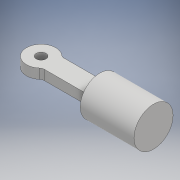
# Autodesk Inventor part: поршень
Saved by Autodesk Inventor 2017.3 (Build 213256000, 256)
## iProperties
Part Number: поршень
Material: Типовые
Document SubType Name: Modeling
Designer: Alexnav
Density: 1 g/cm^3
Appearance: По умолчанию
Mass: 116.064 g
Surface Area: 174.829 cm^2
Volume: 116.064 cm^3
Author: Alexnav
Autodesk Inventor part; units mm, degrees
ref_plane "YZ Plane" through (0, 0, 0) normal (1, 0, 0) x (0, 1, 0)
ref_plane "XZ Plane" through (0, 0, 0) normal (0, 1, 0) x (-1, 0, 0)
ref_plane "XY Plane" through (0, 0, 0) normal (0, 0, 1) x (1, 0, 0)
sketch "Эскиз1" plane through (0, 0, 0) normal (0, 0, 1) x (1, 0, 0)
  line L0 (-12.2268, 10) -> (34.5444, 10)
  line L1 (-55.4556, 0) -> (49.5444, 0) projected
  line L2 (-12.2268, -10) -> (34.5444, -10)
  arc A0 (-15.534, 11.25) -> (-15.534, -11.25) centre (-25.4556, 0) ccw
  circle A1 centre (-25.4556, 0) radius 5
  line L3 (34.5444, 10) -> (34.5444, -10)
  arc A2 (-15.534, 11.25) -> (-12.2268, 10) centre (-12.2268, 15) ccw
  arc A3 (-12.2268, -10) -> (-15.534, -11.25) centre (-12.2268, -15) ccw
  point P0 (0, 0)
  point P1 (-14.2752, 10)
  point P2 (-14.2752, -10)
  dimension "d0" = 15
  dimension "d1" = 20
  dimension "d2" = 10
  dimension "d12" = 5
  dimension "d13" = 60
  constraints: 8 point on circle, 6 end point, 4 centre point, 4 tangent, 3 point on line, 2 horizontal, 1 coincident, 1 equal radius, 1 parallel, 1 perpendicular, 1 other
  measures "d0" radius of A0
  measures "d1" distance between parallel lines of L2 L0
  measures "d2" diameter of A1
  measures "d12" radius of A2
  measures "d13" distance from line of L3 A0.centre
extrude "Выдавливание1" add sketch "Эскиз1" along normal blind 5 and the other way blind 5 contours L0 L3 L1 A1 A0 A2 | L3 L2 A3 A0 L1 A1
sketch "Эскиз4" plane through (0, 0, 0) normal (0, 0, 1) x (1, 0, 0)
  line L0 (-20.9089, 0) -> (125.4533, 0) projected
  line L1 (34.5444, 10) -> (34.5444, -10) projected
  line L2 (34.5444, 0) -> (89.5444, 0)
  line L3 (89.5444, 0) -> (89.5444, 20)
  line L4 (89.5444, 20) -> (34.5444, 20)
  line L5 (34.5444, 20) -> (34.5444, 0)
  point P0 (0, 0)
  dimension "d7" = 40
  dimension "d8" = 55
  constraints: 8 end point, 2 parallel, 1 horizontal, 1 midpoint, 1 perpendicular
  measures "d7" diameter of L4 L0
  measures "d8" distance of L3.end L4.end
revolve "Вращение1" add sketch "Эскиз4" angle 360 about axis through (-10, 0, 0) along (1, 0, 0)
